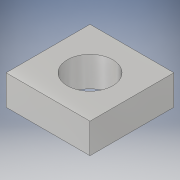
# Autodesk Inventor part: NUT_2MM
Saved by Autodesk Inventor 2017.3 (Build 213256000, 256)
## iProperties
Created: 2018-01-03
Part Number: NUT_2MM
Material: Generic
Document SubType Name: Modeling
Designer: Alex
Density: 1 g/cm^3
Appearance: Aluminum - Polished
nut_A: 4,350 mm
nut_B: 1,550 mm
nut_C: 2,350 mm
Author: Alex
Autodesk Inventor part; units mm, degrees
ref_plane "YZ Plane" through (0, 0, 0) normal (1, 0, 0) x (0, 1, 0)
ref_plane "XZ Plane" through (0, 0, 0) normal (0, 1, 0) x (-1, 0, 0)
ref_plane "XY Plane" through (0, 0, 0) normal (0, 0, 1) x (1, 0, 0)
sketch "Sketch1" plane through (0, 0, 0) normal (0, 1, 0) x (-1, 0, 0)
  line L0 (-2.175, 2.175) -> (2.175, 2.175)
  line L1 (2.175, 2.175) -> (2.175, -2.175)
  line L2 (2.175, -2.175) -> (-2.175, -2.175)
  line L3 (-2.175, -2.175) -> (-2.175, 2.175)
  circle A0 centre (0, 0) radius 1.175
  point P0 (0, 2.175)
  point P1 (2.175, 0)
  dimension "d0" = 4.35
  dimension "d1" = 2.35
  constraints: 8 end point, 2 midpoint, 2 parallel, 2 perpendicular, 1 centre point, 1 coincident, 1 horizontal, 1 horizontal alignment, 1 vertical alignment
  measures "d0" distance of L0.end L1.end
  measures "d1" diameter of A0
extrude "Extrusion1" add sketch "Sketch1" along normal blind 1.55
equation "\"d0\" = nut_A"
equation "\"d1\" = nut_C"
equation "\"d2\" = nut_B"
equation "\"nut_A\" = 4.35"
equation "\"nut_C\" = 2.35"
equation "\"nut_B\" = 1.55"
body "Solid1"
